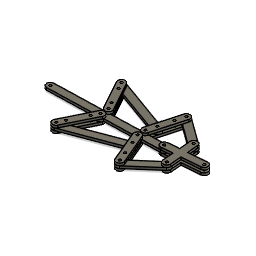
1-DOF v15 (Autodesk Fusion 360 design; units mm, degrees)
Autodesk Fusion 360 part; units mm, degrees
sketch "handle" plane through (0, 0, 0) normal (0, 0, 1) x (1, 0, 0)
  line L0 (-25, 5) -> (-25, -5) construction
  line L1 (25, -5) -> (25, 5) construction
  line L2 (25, 5) -> (-25, -5) construction
  line L3 (-25, 5) -> (25, -5) construction
  arc A0 (25, -5) -> (25, 5) centre (25, 0) ccw
  arc A1 (-25, 5) -> (-25, -5) centre (-25, 0) ccw
  line L4 (-25, 0) -> (25, 0) construction
  line L5 (0, 20) -> (-10, 20) construction
  line L6 (-10, -20) -> (0, -20) construction
  line L7 (0, 20) -> (-10, -20) construction
  line L8 (-10, 20) -> (0, -20) construction
  arc A2 (0, 20) -> (-10, 20) centre (-5, 20) ccw
  arc A3 (-10, -20) -> (0, -20) centre (-5, -20) ccw
  circle A4 centre (-25, 0) radius 1.6
  circle A5 centre (-5, 20) radius 1.6
  circle A6 centre (-5, -20) radius 1.6
  circle A7 centre (25, 0) radius 1.6
  line L9 (25, 5) -> (0, 5)
  line L10 (-10, 5) -> (-25, 5)
  line L11 (-25, -5) -> (-10, -5)
  line L12 (0, -5) -> (25, -5)
  line L13 (0, -20) -> (0, -5)
  line L14 (0, 5) -> (0, 20)
  line L15 (-10, 20) -> (-10, 5)
  line L16 (-10, -5) -> (-10, -20)
  line L17 (0, 5) -> (0, -5) construction
  point P0 (-5, 0)
  dimension "d1" = 50
  dimension "link_width" = 10
  dimension "d3" = 10
  dimension "handle_T_width" = 40
  dimension "handle_T_height" = 20
  dimension "joint_hole_size" = 3.2
  dimension "d7" = 3.2
  dimension "d8" = 3.2
  dimension "d9" = 3.2
  constraint perpendicular L0 L9
  constraint parallel L9 L11
  constraint parallel L0 L1
  constraint horizontal L9
  constraint coincident L2 origin
  constraint coincident L3 origin
  constraint midpoint L1 A0.centre
  constraint midpoint L0 A1.centre
  constraint tangent A1 L9
  constraint coincident A1.centre L4.start
  constraint coincident A0.centre L4.end
  constraint perpendicular L5 L15
  constraint parallel L5 L6
  constraint parallel L13 L15
  constraint horizontal L5
  constraint coincident L7 P0
  constraint coincident L8 P0
  constraint coincident L4 P0
  constraint midpoint L5 A2.centre
  constraint midpoint L6 A3.centre
  constraint tangent A3 L15
  constraint concentric A1 A4
  constraint concentric A2 A5
  constraint concentric A3 A6
  constraint concentric A0 A7
  constraint collinear L9 L10
  constraint coincident L9.end L13
  constraint collinear L11 L12
  constraint coincident L11.end L15
  constraint collinear L13 L14
  constraint collinear L15 L16
  constraint coincident L9 L14.start
  constraint coincident L12 L13.end
  constraint perpendicular L12 L17
  constraint coincident origin L17
  measures "d1" distance of L0.end L1.start L1.end
  measures "link_width" distance of L0.start L0.end
  measures "d3" distance of L6.start L6.end
  measures "handle_T_width" distance of L5.end L6.start
  measures "handle_T_height" distance of A1.centre P0
  measures "joint_hole_size" diameter of A4
  measures "d7" diameter of A5
  measures "d8" diameter of A6
  measures "d9" diameter of A7
extrude "Extrude1" add sketch "handle" along normal blind 3.2 makes body 1
sketch "base" plane through (0, 0, 0) normal (0, 0, 1) x (1, 0, 0)
  line L0 (75, 5) -> (75, -5) construction
  line L1 (-75, -5) -> (-75, 5) construction
  line L2 (-75, 5) -> (75, -5) construction
  line L3 (75, 5) -> (-75, -5) construction
  arc A0 (-75, 5) -> (-75, -5) centre (-75, 0) ccw
  arc A1 (75, -5) -> (75, 5) centre (75, 0) ccw
  line L4 (-40, -5.5) -> (-50, -5.5) construction
  line L5 (-50, 5.5) -> (-40, 5.5) construction
  line L6 (-40, -5.5) -> (-50, 5.5) construction
  line L7 (-50, -5.5) -> (-40, 5.5) construction
  arc A2 (-40, 5.5) -> (-50, 5.5) centre (-45, 5.5) ccw
  arc A3 (-50, -5.5) -> (-40, -5.5) centre (-45, -5.5) ccw
  line L8 (-75, 5) -> (-50, 5)
  line L9 (-50, -5) -> (-75, -5)
  line L10 (-50, -5.5) -> (-50, -5)
  line L11 (-50, 5) -> (-50, 5.5)
  line L12 (-40, -5) -> (-40, -5.5)
  line L13 (-40, 5.5) -> (-40, 5)
  circle A4 centre (-45, 5.5) radius 1.6
  circle A5 centre (-75, 0) radius 1.6
  circle A6 centre (-45, -5.5) radius 1.6
  circle A7 centre (75, 0) radius 1.6
  line L14 (10.0183, 3.8997) -> (0.0183, 3.8997) construction
  line L15 (0.0183, -7.1003) -> (10.0183, -7.1003) construction
  line L16 (10.0183, 3.8997) -> (0.0183, -7.1003) construction
  line L17 (0.0183, 3.8997) -> (10.0183, -7.1003) construction
  arc A8 (0.0183, -7.1003) -> (10.0183, -7.1003) centre (5.0183, -7.1003) ccw
  arc A9 (10.0183, 3.8997) -> (0.0183, 3.8997) centre (5.0183, 3.8997) ccw
  line L18 (-40, 5) -> (0.0183, 5)
  line L19 (10.0183, 5) -> (75, 5)
  line L20 (75, -5) -> (10.0183, -5)
  line L21 (0.0183, -5) -> (-40, -5)
  line L22 (10.0183, 5) -> (10.0183, 3.8997)
  line L23 (10.0183, -7.1003) -> (10.0183, -5)
  line L24 (0.0183, -5) -> (0.0183, -7.1003)
  line L25 (0.0183, 3.8997) -> (0.0183, 5)
  line L26 (75, 0) -> (-75, 0) construction
  circle A10 centre (5.0183, 3.8997) radius 1.6
  circle A11 centre (5.0183, -7.1003) radius 1.6
  point P0 (-45, 0)
  point P1 (5.0183, -1.6003)
  dimension "d12" = 10
  dimension "d13" = 150
  dimension "d14" = 10
  dimension "base_T_width" = 11
  dimension "d17" = 3.2
  dimension "d18" = 3.2
  dimension "d19" = 3.2
  dimension "d20" = 3.2
  dimension "base_T_height" = 30
  dimension "d210" = 10
  dimension "lever_attach_width" = 11
  dimension "lever_height" = 70
  dimension "d213" = 3.2
  dimension "d214" = 3.2
  constraint perpendicular L0 L8
  constraint parallel L8 L20
  constraint parallel L0 L1
  constraint horizontal L8
  constraint coincident L2 origin
  constraint coincident L3 origin
  constraint midpoint L0 A1.centre
  constraint midpoint L1 A0.centre
  constraint tangent A0 L8
  constraint perpendicular L4 L10
  constraint parallel L4 L5
  constraint parallel L10 L13
  constraint horizontal L4
  constraint coincident L6 P0
  constraint coincident L7 P0
  constraint midpoint L5 A2.centre
  constraint midpoint L4 A3.centre
  constraint tangent A3 L13
  constraint collinear L8 L18
  constraint coincident L8.end L10
  constraint coincident L12.start L13
  constraint collinear L9 L20
  constraint collinear L10 L11
  constraint collinear L12 L13
  constraint concentric A2 A4
  constraint concentric A0 A5
  constraint concentric A3 A6
  constraint concentric A1 A7
  constraint perpendicular L14 L25
  constraint parallel L14 L15
  constraint parallel L23 L25
  constraint horizontal L14
  constraint coincident L16 P1
  constraint coincident L17 P1
  constraint midpoint L14 A9.centre
  constraint midpoint L15 A8.centre
  constraint tangent A8 L25
  constraint coincident L19.start L23
  constraint collinear L18 L19
  constraint collinear L20 L21
  constraint coincident L21.start L25
  constraint collinear L22 L23
  constraint collinear L24 L25
  constraint coincident A1.centre A7.centre
  constraint coincident A0.centre A5.centre
  constraint coincident P0 L26
  constraint concentric A9 A10
  constraint concentric A8 A11
  measures "d12" distance of L0.start L0.end
  measures "d13" distance of L0.end L1.start
  measures "d14" distance of L5.start L5.end
  measures "base_T_width" distance of L4.end L5.start
  measures "d17" diameter of A4
  measures "d18" diameter of A5
  measures "d19" diameter of A6
  measures "d20" diameter of A7
  measures "base_T_height" horizontal distance of A2.centre A0.centre
  measures "d210" distance of L15.start L15.end
  measures "lever_attach_width" distance of L14.end L15.start
  measures "lever_height" distance of A1.centre P1
  measures "d213" diameter of A10
  measures "d214" diameter of A11
extrude "Extrude2" add sketch "base" along normal blind 3.2 separate body makes body 2
copy_body "Body->Comp1" bodies 1 removing the originals makes body 3 in component "handle"
copy_body "Body->Comp3" bodies 2 removing the originals makes body 4 in component "base"
sketch "handle_link" plane through (0, 0, 0) normal (0, 0, 1) x (1, 0, 0)
  line L0 (-22.5, 5) -> (22.5, 5)
  line L1 (22.5, 5) -> (22.5, -5) construction
  line L2 (22.5, -5) -> (-22.5, -5)
  line L3 (-22.5, -5) -> (-22.5, 5) construction
  line L4 (-22.5, 5) -> (22.5, -5) construction
  line L5 (22.5, 5) -> (-22.5, -5) construction
  arc A0 (22.5, -5) -> (22.5, 5) centre (22.5, 0) ccw
  arc A1 (-22.5, 5) -> (-22.5, -5) centre (-22.5, 0) ccw
  circle A2 centre (22.5, 0) radius 1.6
  circle A3 centre (-22.5, 0) radius 1.6
  dimension "handle_link_length" = 45
  dimension "d48" = 10
  dimension "d49" = 3.2
  dimension "d50" = 3.2
  constraint perpendicular L0 L1
  constraint parallel L0 L2
  constraint parallel L1 L3
  constraint horizontal L0
  constraint coincident L4 origin
  constraint coincident L5 origin
  constraint midpoint L1 A0.centre
  constraint midpoint L3 A1.centre
  constraint tangent L0 A1
  constraint concentric A0 A2
  constraint concentric A1 A3
  measures "handle_link_length" distance of L1.end L2.end
  measures "d48" distance of L0.end L1.end
  measures "d49" diameter of A2
  measures "d50" diameter of A3
extrude "Extrude3" add sketch "handle_link" along normal blind 3.2 separate body makes body 5
copy_body "Body->Comp4" bodies 5 removing the originals makes body 6 in component "handle_link"
sketch "base_link" plane through (0, 0, 0) normal (0, 0, 1) x (1, 0, 0)
  line L0 (22.5, 5) -> (-22.5, 5)
  line L1 (-22.5, 5) -> (-22.5, -5) construction
  line L2 (-22.5, -5) -> (22.5, -5)
  line L3 (22.5, -5) -> (22.5, 5) construction
  line L4 (22.5, 5) -> (-22.5, -5) construction
  line L5 (-22.5, 5) -> (22.5, -5) construction
  arc A0 (-22.5, 5) -> (-22.5, -5) centre (-22.5, 0) ccw
  arc A1 (22.5, -5) -> (22.5, 5) centre (22.5, 0) ccw
  circle A2 centre (-22.5, 0) radius 1.6
  circle A3 centre (22.5, 0) radius 1.6
  line L6 (0, 5) -> (0, -5) construction
  line L7 (-22.5, 0) -> (22.5, 0) construction
  circle A4 centre (-9.5, 0) radius 1.6
  circle A5 centre (9.5, 0) radius 1.6
  dimension "d104" = 10
  dimension "base_link_length" = 45
  dimension "d106" = 3.2
  dimension "d107" = 3.2
  dimension "d208" = 3.2
  dimension "lever_attach" = 13
  constraint perpendicular L0 L1
  constraint parallel L0 L2
  constraint parallel L1 L3
  constraint horizontal L0
  constraint coincident L4 origin
  constraint coincident L5 origin
  constraint midpoint L1 A0.centre
  constraint midpoint L3 A1.centre
  constraint tangent L0 A1
  constraint concentric A0 A2
  constraint concentric A1 A3
  constraint midpoint L0 L6.start
  constraint midpoint L2 L6.end
  constraint coincident A0.centre A2.centre
  constraint coincident A1.centre A3.centre
  constraint coincident L7 A4.centre
  constraint symmetric L6 A4 A5
  measures "d104" distance of L0.start L2.end
  measures "base_link_length" distance of L1 L3
  measures "d106" diameter of A2
  measures "d107" diameter of A3
  measures "d208" diameter of A4
  measures "lever_attach" distance of A0.centre A4.centre
extrude "Extrude4" add sketch "base_link" along normal blind 3.2 separate body makes body 7
copy_body "Body->Comp5" bodies 7 removing the originals makes body 8 in component "base_link"
sketch "lever_low" plane through (0, 0, 0) normal (0, 1, 0) x (1, 0, 0)
  line L0 (22.5, 5) -> (-22.5, 5)
  line L1 (-22.5, 5) -> (-22.5, -5) construction
  line L2 (-22.5, -5) -> (22.5, -5)
  line L3 (22.5, -5) -> (22.5, 5) construction
  line L4 (22.5, 5) -> (-22.5, -5) construction
  line L5 (-22.5, 5) -> (22.5, -5) construction
  arc A0 (-22.5, 5) -> (-22.5, -5) centre (-22.5, 0) ccw
  arc A1 (22.5, -5) -> (22.5, 5) centre (22.5, 0) ccw
  circle A2 centre (-22.5, 0) radius 1.6
  circle A3 centre (22.5, 0) radius 1.6
  circle A4 centre (-12.5, 0) radius 1.6
  line L6 (0, 5) -> (0, -5) construction
  line L7 (-22.5, 0) -> (22.5, 0) construction
  circle A5 centre (12.5, 0) radius 1.6
  dimension "lever_low_length" = 45
  dimension "d216" = 10
  dimension "d217" = 3.2
  dimension "d218" = 3.2
  dimension "d219" = 3.2
  dimension "lever_tendon_length" = 10
  constraint perpendicular L0 L1
  constraint parallel L0 L2
  constraint parallel L1 L3
  constraint horizontal L0
  constraint coincident L4 origin
  constraint coincident L5 origin
  constraint midpoint L1 A0.centre
  constraint midpoint L3 A1.centre
  constraint tangent L0 A1
  constraint concentric A0 A2
  constraint concentric A1 A3
  constraint midpoint L0 L6.start
  constraint midpoint L2 L6.end
  constraint coincident A0.centre A2.centre
  constraint coincident A1.centre A3.centre
  constraint coincident A4.centre L7
  constraint symmetric A4 L6 A5
  measures "lever_low_length" distance of L1.end L2.end
  measures "d216" distance of L0.end L1.end
  measures "d217" diameter of A2
  measures "d218" diameter of A3
  measures "d219" diameter of A4
  measures "lever_tendon_length" distance of A0.centre A4.centre
extrude "Extrude5" add sketch "lever_low" along normal blind 3.2 separate body makes body 9
copy_body "Body->Comp6" bodies 9 removing the originals makes body 10 in component "low_lever"
sketch "lever_high" plane through (0, 0, 0) normal (0, 1, 0) x (1, 0, 0)
  line L0 (40, 5) -> (-40, 5)
  line L1 (-40, 5) -> (-40, -5) construction
  line L2 (-40, -5) -> (40, -5)
  line L3 (40, -5) -> (40, 5) construction
  line L4 (40, 5) -> (-40, -5) construction
  line L5 (-40, 5) -> (40, -5) construction
  arc A0 (-40, 5) -> (-40, -5) centre (-40, 0) ccw
  arc A1 (40, -5) -> (40, 5) centre (40, 0) ccw
  circle A2 centre (-40, 0) radius 1.6
  circle A3 centre (40, 0) radius 1.6
  dimension "d224" = 10
  dimension "lever_high_length" = 80
  dimension "d226" = 3.2
  dimension "d227" = 3.2
  constraint perpendicular L0 L1
  constraint parallel L0 L2
  constraint parallel L1 L3
  constraint horizontal L0
  constraint coincident L4 origin
  constraint coincident L5 origin
  constraint midpoint L1 A0.centre
  constraint midpoint L3 A1.centre
  constraint tangent L0 A1
  constraint concentric A0 A2
  constraint concentric A1 A3
  measures "d224" distance of L0.end L1.end
  measures "lever_high_length" distance of L1.end L2.end
  measures "d226" diameter of A2
  measures "d227" diameter of A3
extrude "Extrude6" add sketch "lever_high" along normal blind 3.2 separate body makes body 11
copy_body "Body->Comp7" bodies 11 removing the originals makes body 12 in component "lever_high"
sketch "Sketch7" plane through (0, 0, 0) normal (1, 0, 0) x (0, 0, -1)
  line L0 (-19, 18) -> (-13, 18)
  line L1 (-13, 18) -> (-13, 12)
  line L2 (-13, 12) -> (-19, 12)
  line L3 (-19, 12) -> (-19, 18)
  line L4 (-18, 17) -> (-14, 17)
  line L5 (-14, 17) -> (-14, 13)
  line L6 (-14, 13) -> (-18, 13)
  line L7 (-18, 13) -> (-18, 17)
  constraint horizontal L0
  constraint vertical L1
  constraint horizontal L2
  constraint vertical L3
  constraint horizontal L4
  constraint vertical L5
  constraint horizontal L6
  constraint vertical L7
sketch "Sketch8" plane through (0, 0, 0) normal (0, 1, 0) x (1, 0, 0)
component "handle" placed x (0.99961, 0, -0.027924) y (-0.027924, 0, -0.99961) z (0, 1, 0) at (-0.0097, 1.6, 2.7019)
component "base" placed x (-0.99961, 0, 0.027924) y (0.027924, 0, 0.99961) z (0, 1, 0) at (-99.9708, -1.6, 5.4943)
component "handle" placed x (0.99961, 0, -0.027924) y (-0.027924, 0, -0.99961) z (0, 1, 0) at (-0.0097, -4.8, 2.7019)
component "handle_link" placed x (0.799827, 0, 0.600231) y (0.600231, 0, -0.799827) z (0, 1, 0) at (-23.5624, -1.6, -30.6559)
component "handle_link" placed x (0.76507, 0, -0.643947) y (-0.643947, 0, -0.76507) z (0, 1, 0) at (-21.6634, -1.6, 37.3225)
component "base_link" placed x (0.301853, 0, -0.953354) y (-0.953354, 0, -0.301853) z (0, 1, 0) at (-48.3502, -4.8, -22.7106)
component "base_link" placed x (0.301853, 0, -0.953354) y (-0.953354, 0, -0.301853) z (0, 1, 0) at (-48.3502, 1.6, -22.7106)
component "base_link" placed x (0.354605, 0, 0.935016) y (0.935016, 0, -0.354605) z (0, 1, 0) at (-46.8561, 1.6, 30.7735)
component "base_link" placed x (0.354605, 0, 0.935016) y (0.935016, 0, -0.354605) z (0, 1, 0) at (-46.8561, -4.8, 30.7735)
component "low_lever" placed x (-0.452752, 0, 0.891636) y (0, 1, 0) z (-0.891636, 0, -0.452752) at (-115.0651, 1.6, 29.5944)
component "low_lever" placed x (-0.452752, 0, 0.891636) y (0, 1, 0) z (-0.891636, 0, -0.452752) at (-115.0651, -4.8, 29.5944)
component "lever_high" placed x (0.93784, 0, -0.347068) y (0, 1, 0) z (0.347068, 0, 0.93784) at (-87.7384, -1.6, 35.7735)
component "low_lever" placed x (-0.469905, 0, -0.882717) y (0, -1, 0) z (-0.882717, 0, 0.469905) at (-115.7582, 4.8, -21.3242)
component "low_lever" placed x (-0.469905, 0, -0.882717) y (0, -1, 0) z (-0.882717, 0, 0.469905) at (-115.7582, -1.6, -21.3242)
component "lever_high" placed x (0.938916, 0, 0.344145) y (0, -1, 0) z (0.344145, 0, -0.938916) at (-88.7744, 1.6, -27.4195)
equation "d7 = joint_hole_size"
equation "d8 = joint_hole_size"
equation "d9 = joint_hole_size"
equation "thickness = 3.2 mm"
equation "d12 = link_width"
equation "d14 = link_width"
equation "d17 = joint_hole_size"
equation "d18 = joint_hole_size"
equation "d19 = joint_hole_size"
equation "d20 = joint_hole_size"
equation "d21 = thickness"
equation "d48 = link_width"
equation "d49 = joint_hole_size"
equation "d50 = joint_hole_size"
equation "d51 = thickness"
equation "d104 = link_width"
equation "d106 = joint_hole_size"
equation "d107 = joint_hole_size"
equation "d108 = thickness"
equation "d208 = joint_hole_size"
equation "d210 = link_width"
equation "d213 = joint_hole_size"
equation "d214 = joint_hole_size"
equation "d216 = link_width"
equation "d217 = joint_hole_size"
equation "d218 = joint_hole_size"
equation "d219 = joint_hole_size"
equation "d221 = thickness"
equation "d224 = link_width"
equation "d226 = joint_hole_size"
equation "d227 = joint_hole_size"
equation "d228 = thickness"
named bodies: "base", "handle", "handle_link", "base_link", "low_lever", "lever_high"
